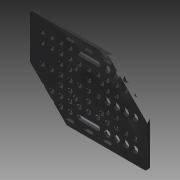
# Autodesk Inventor part: 80mm gantry plate
Saved by Autodesk Inventor 2014 SP1 (Build 180222100, 222)
## iProperties
Created: 2016-04-10
Part Number: 80mm gantry plate
Material: Generic
Document SubType Name: Modeling
Designer: Ben
Density: 1 g/cm^3
Appearance: Default
Author: Ben
Autodesk Inventor part; units mm, degrees
ref_plane "YZ Plane" through (0, 0, 0) normal (1, 0, 0) x (0, 1, 0)
ref_plane "XZ Plane" through (0, 0, 0) normal (0, 1, 0) x (-1, 0, 0)
ref_plane "XY Plane" through (0, 0, 0) normal (0, 0, 1) x (1, 0, 0)
sketch "Sketch1" plane through (0, 0, 0) normal (0, 0, 1) x (1, 0, 0)
  line L0 (-63.5, 44) -> (63.5, 44)
  line L1 (63.5, 44) -> (63.5, -44)
  line L2 (63.5, -44) -> (-63.5, -44)
  line L3 (-63.5, -44) -> (-63.5, 44)
  line L4 (0, 44) -> (0, -44) construction
  line L5 (-63.5, 0) -> (63.5, 0) construction
  point P0 (0, 0)
  dimension "d0" = 127
  dimension "d1" = 88
  constraints: 12 end point, 6 midpoint, 2 parallel, 1 horizontal, 1 perpendicular
  measures "d0" distance of L1.end L2.end
  measures "d1" distance of L0.end L1.end
extrude "Extrusion1" add sketch "Sketch1" along normal blind 3
sketch "Sketch2" plane through (0, 0, 3) normal (0, 0, 1) x (1, 0, 0)
  line L0 (-63.5, -44) -> (63.5, -44) projected
  line L1 (63.5, -44) -> (63.5, 44) projected
  circle A0 centre (0, 0) radius 2.5
  line L2 (0, 0) -> (78.1267, 0) construction
  line L3 (0, 0) -> (0, 59.5743) construction
  circle A1 centre (10, 0) radius 2.5
  circle A2 centre (20, 0) radius 2.5
  circle A3 centre (30, 0) radius 2.5
  circle A4 centre (40, 0) radius 2.5
  circle A5 centre (50, 0) radius 2.5
  circle A6 centre (-10, 0) radius 2.5
  circle A7 centre (0, 0) radius 2.5
  circle A8 centre (10, 0) radius 2.5
  circle A9 centre (20, 0) radius 2.5
  circle A10 centre (30, 0) radius 2.5
  circle A11 centre (40, 0) radius 2.5
  circle A12 centre (-20, 0) radius 2.5
  circle A13 centre (-10, 0) radius 2.5
  circle A14 centre (0, 0) radius 2.5
  circle A15 centre (10, 0) radius 2.5
  circle A16 centre (20, 0) radius 2.5
  circle A17 centre (30, 0) radius 2.5
  circle A18 centre (-30, 0) radius 2.5
  circle A19 centre (-20, 0) radius 2.5
  circle A20 centre (-10, 0) radius 2.5
  circle A21 centre (0, 0) radius 2.5
  circle A22 centre (10, 0) radius 2.5
  circle A23 centre (20, 0) radius 2.5
  circle A24 centre (-40, 0) radius 2.5
  circle A25 centre (-30, 0) radius 2.5
  circle A26 centre (-20, 0) radius 2.5
  circle A27 centre (-10, 0) radius 2.5
  circle A28 centre (0, 0) radius 2.5
  circle A29 centre (10, 0) radius 2.5
  circle A30 centre (-50, 0) radius 2.5
  circle A31 centre (-40, 0) radius 2.5
  circle A32 centre (-30, 0) radius 2.5
  circle A33 centre (-20, 0) radius 2.5
  circle A34 centre (-10, 0) radius 2.5
  circle A35 centre (0, 0) radius 2.5
  circle A36 centre (0, 20) radius 2.5
  circle A37 centre (10, 20) radius 2.5
  circle A38 centre (20, 20) radius 2.5
  circle A39 centre (30, 20) radius 2.5
  circle A40 centre (40, 20) radius 2.5
  circle A41 centre (50, 20) radius 2.5
  circle A42 centre (-10, 20) radius 2.5
  circle A43 centre (0, 20) radius 2.5
  circle A44 centre (10, 20) radius 2.5
  circle A45 centre (20, 20) radius 2.5
  circle A46 centre (30, 20) radius 2.5
  circle A47 centre (40, 20) radius 2.5
  circle A48 centre (-20, 20) radius 2.5
  circle A49 centre (-10, 20) radius 2.5
  circle A50 centre (0, 20) radius 2.5
  circle A51 centre (10, 20) radius 2.5
  circle A52 centre (20, 20) radius 2.5
  circle A53 centre (30, 20) radius 2.5
  circle A54 centre (-30, 20) radius 2.5
  circle A55 centre (-20, 20) radius 2.5
  circle A56 centre (-10, 20) radius 2.5
  circle A57 centre (0, 20) radius 2.5
  circle A58 centre (10, 20) radius 2.5
  circle A59 centre (20, 20) radius 2.5
  circle A60 centre (-40, 20) radius 2.5
  circle A61 centre (-30, 20) radius 2.5
  circle A62 centre (-20, 20) radius 2.5
  circle A63 centre (-10, 20) radius 2.5
  circle A64 centre (0, 20) radius 2.5
  circle A65 centre (10, 20) radius 2.5
  circle A66 centre (-50, 20) radius 2.5
  circle A67 centre (-40, 20) radius 2.5
  circle A68 centre (-30, 20) radius 2.5
  circle A69 centre (-20, 20) radius 2.5
  circle A70 centre (-10, 20) radius 2.5
  circle A71 centre (0, 20) radius 2.5
  circle A72 centre (0, -20) radius 2.5
  circle A73 centre (10, -20) radius 2.5
  circle A74 centre (20, -20) radius 2.5
  circle A75 centre (30, -20) radius 2.5
  circle A76 centre (40, -20) radius 2.5
  circle A77 centre (50, -20) radius 2.5
  circle A78 centre (-10, -20) radius 2.5
  circle A79 centre (0, -20) radius 2.5
  circle A80 centre (10, -20) radius 2.5
  circle A81 centre (20, -20) radius 2.5
  circle A82 centre (30, -20) radius 2.5
  circle A83 centre (40, -20) radius 2.5
  circle A84 centre (-20, -20) radius 2.5
  circle A85 centre (-10, -20) radius 2.5
  circle A86 centre (0, -20) radius 2.5
  circle A87 centre (10, -20) radius 2.5
  circle A88 centre (20, -20) radius 2.5
  circle A89 centre (30, -20) radius 2.5
  circle A90 centre (-30, -20) radius 2.5
  circle A91 centre (-20, -20) radius 2.5
  circle A92 centre (-10, -20) radius 2.5
  circle A93 centre (0, -20) radius 2.5
  circle A94 centre (10, -20) radius 2.5
  circle A95 centre (20, -20) radius 2.5
  circle A96 centre (-40, -20) radius 2.5
  circle A97 centre (-30, -20) radius 2.5
  circle A98 centre (-20, -20) radius 2.5
  circle A99 centre (-10, -20) radius 2.5
  circle A100 centre (0, -20) radius 2.5
  circle A101 centre (10, -20) radius 2.5
  circle A102 centre (-50, -20) radius 2.5
  circle A103 centre (-40, -20) radius 2.5
  circle A104 centre (-30, -20) radius 2.5
  circle A105 centre (-20, -20) radius 2.5
  circle A106 centre (-10, -20) radius 2.5
  circle A107 centre (0, -20) radius 2.5
  circle A108 centre (0, 0) radius 2.5
  circle A109 centre (10, 0) radius 2.5
  circle A110 centre (20, 0) radius 2.5
  circle A111 centre (30, 0) radius 2.5
  circle A112 centre (40, 0) radius 2.5
  circle A113 centre (50, 0) radius 2.5
  circle A114 centre (-10, 0) radius 2.5
  circle A115 centre (0, 0) radius 2.5
  circle A116 centre (10, 0) radius 2.5
  circle A117 centre (20, 0) radius 2.5
  circle A118 centre (30, 0) radius 2.5
  circle A119 centre (40, 0) radius 2.5
  circle A120 centre (-20, 0) radius 2.5
  circle A121 centre (-10, 0) radius 2.5
  circle A122 centre (0, 0) radius 2.5
  circle A123 centre (10, 0) radius 2.5
  circle A124 centre (20, 0) radius 2.5
  circle A125 centre (30, 0) radius 2.5
  circle A126 centre (-30, 0) radius 2.5
  circle A127 centre (-20, 0) radius 2.5
  circle A128 centre (-10, 0) radius 2.5
  circle A129 centre (0, 0) radius 2.5
  circle A130 centre (10, 0) radius 2.5
  circle A131 centre (20, 0) radius 2.5
  circle A132 centre (-40, 0) radius 2.5
  circle A133 centre (-30, 0) radius 2.5
  circle A134 centre (-20, 0) radius 2.5
  circle A135 centre (-10, 0) radius 2.5
  circle A136 centre (0, 0) radius 2.5
  circle A137 centre (10, 0) radius 2.5
  circle A138 centre (-50, 0) radius 2.5
  circle A139 centre (-40, 0) radius 2.5
  circle A140 centre (-30, 0) radius 2.5
  circle A141 centre (-20, 0) radius 2.5
  circle A142 centre (-10, 0) radius 2.5
  circle A143 centre (0, 0) radius 2.5
  circle A144 centre (-14.1421, -14.1421) radius 2.5
  circle A145 centre (0, -20) radius 2.5
  circle A146 centre (14.1421, -14.1421) radius 2.5
  circle A147 centre (20, 0) radius 2.5
  circle A148 centre (14.1421, 14.1421) radius 2.5
  circle A149 centre (0, 20) radius 2.5
  circle A150 centre (-14.1421, 14.1421) radius 2.5
  circle A151 centre (0, -10) radius 2.5
  circle A152 centre (10, 0) radius 2.5
  circle A153 centre (0, 10) radius 2.5
  circle A154 centre (-20, 10) radius 2.5
  circle A155 centre (-30, 10) radius 2.5
  circle A156 centre (-20, 10) radius 2.5
  circle A157 centre (-30, 10) radius 2.5
  circle A158 centre (-20, 10) radius 2.5
  circle A159 centre (-30, 10) radius 2.5
  circle A160 centre (-20, 10) radius 2.5
  circle A161 centre (-20, 10) radius 2.5
  circle A162 centre (-30, 10) radius 2.5
  circle A163 centre (-20, 10) radius 2.5
  circle A164 centre (-20, 10) radius 2.5
  circle A165 centre (-20, 10) radius 2.5
  circle A166 centre (-30, 10) radius 2.5
  circle A167 centre (-30, 10) radius 2.5
  circle A168 centre (-20, 20) radius 2.5
  circle A169 centre (-30, 20) radius 2.5
  circle A170 centre (-20, 20) radius 2.5
  circle A171 centre (-30, 20) radius 2.5
  circle A172 centre (-20, 20) radius 2.5
  circle A173 centre (-30, 20) radius 2.5
  circle A174 centre (-20, 20) radius 2.5
  circle A175 centre (-20, 20) radius 2.5
  circle A176 centre (-30, 20) radius 2.5
  circle A177 centre (-20, 20) radius 2.5
  circle A178 centre (-20, 20) radius 2.5
  circle A179 centre (-20, 20) radius 2.5
  circle A180 centre (-30, 20) radius 2.5
  circle A181 centre (-30, 20) radius 2.5
  circle A182 centre (-20, 30) radius 2.5
  circle A183 centre (-30, 30) radius 2.5
  circle A184 centre (-20, 30) radius 2.5
  circle A185 centre (-30, 30) radius 2.5
  circle A186 centre (-20, 30) radius 2.5
  circle A187 centre (-30, 30) radius 2.5
  circle A188 centre (-20, 30) radius 2.5
  circle A189 centre (-20, 30) radius 2.5
  circle A190 centre (-30, 30) radius 2.5
  circle A191 centre (-20, 30) radius 2.5
  circle A192 centre (-20, 30) radius 2.5
  circle A193 centre (-20, 30) radius 2.5
  circle A194 centre (-30, 30) radius 2.5
  circle A195 centre (-30, 30) radius 2.5
  circle A196 centre (-20, -10) radius 2.5
  circle A197 centre (-30, -10) radius 2.5
  circle A198 centre (-20, -10) radius 2.5
  circle A199 centre (-30, -10) radius 2.5
  circle A200 centre (-20, -10) radius 2.5
  circle A201 centre (-30, -10) radius 2.5
  circle A202 centre (-20, -10) radius 2.5
  circle A203 centre (-20, -10) radius 2.5
  circle A204 centre (-30, -10) radius 2.5
  circle A205 centre (-20, -10) radius 2.5
  circle A206 centre (-20, -10) radius 2.5
  circle A207 centre (-20, -10) radius 2.5
  circle A208 centre (-30, -10) radius 2.5
  circle A209 centre (-30, -10) radius 2.5
  circle A210 centre (-20, 0) radius 2.5
  circle A211 centre (-30, 0) radius 2.5
  circle A212 centre (-20, 0) radius 2.5
  circle A213 centre (-30, 0) radius 2.5
  circle A214 centre (-20, 0) radius 2.5
  circle A215 centre (-30, 0) radius 2.5
  circle A216 centre (-20, 0) radius 2.5
  circle A217 centre (-20, 0) radius 2.5
  circle A218 centre (-30, 0) radius 2.5
  circle A219 centre (-20, 0) radius 2.5
  circle A220 centre (-20, 0) radius 2.5
  circle A221 centre (-20, 0) radius 2.5
  circle A222 centre (-30, 0) radius 2.5
  circle A223 centre (-30, 0) radius 2.5
  circle A224 centre (-20, 10) radius 2.5
  circle A225 centre (-30, 10) radius 2.5
  circle A226 centre (-20, 10) radius 2.5
  circle A227 centre (-30, 10) radius 2.5
  circle A228 centre (-20, 10) radius 2.5
  circle A229 centre (-30, 10) radius 2.5
  circle A230 centre (-20, 10) radius 2.5
  circle A231 centre (-20, 10) radius 2.5
  circle A232 centre (-30, 10) radius 2.5
  circle A233 centre (-20, 10) radius 2.5
  circle A234 centre (-20, 10) radius 2.5
  circle A235 centre (-20, 10) radius 2.5
  circle A236 centre (-30, 10) radius 2.5
  circle A237 centre (-30, 10) radius 2.5
  circle A238 centre (-20, 20) radius 2.5
  circle A239 centre (-30, 20) radius 2.5
  circle A240 centre (-20, 20) radius 2.5
  circle A241 centre (-30, 20) radius 2.5
  circle A242 centre (-20, 20) radius 2.5
  circle A243 centre (-30, 20) radius 2.5
  circle A244 centre (-20, 20) radius 2.5
  circle A245 centre (-20, 20) radius 2.5
  circle A246 centre (-30, 20) radius 2.5
  circle A247 centre (-20, 20) radius 2.5
  circle A248 centre (-20, 20) radius 2.5
  circle A249 centre (-20, 20) radius 2.5
  circle A250 centre (-30, 20) radius 2.5
  circle A251 centre (-30, 20) radius 2.5
  circle A252 centre (-20, -20) radius 2.5
  circle A253 centre (-30, -20) radius 2.5
  circle A254 centre (-20, -20) radius 2.5
  circle A255 centre (-30, -20) radius 2.5
  circle A256 centre (-20, -20) radius 2.5
  circle A257 centre (-30, -20) radius 2.5
  circle A258 centre (-20, -20) radius 2.5
  circle A259 centre (-20, -20) radius 2.5
  circle A260 centre (-30, -20) radius 2.5
  circle A261 centre (-20, -20) radius 2.5
  circle A262 centre (-20, -20) radius 2.5
  circle A263 centre (-20, -20) radius 2.5
  circle A264 centre (-30, -20) radius 2.5
  circle A265 centre (-30, -20) radius 2.5
  circle A266 centre (-20, -10) radius 2.5
  circle A267 centre (-30, -10) radius 2.5
  circle A268 centre (-20, -10) radius 2.5
  circle A269 centre (-30, -10) radius 2.5
  circle A270 centre (-20, -10) radius 2.5
  circle A271 centre (-30, -10) radius 2.5
  circle A272 centre (-20, -10) radius 2.5
  circle A273 centre (-20, -10) radius 2.5
  circle A274 centre (-30, -10) radius 2.5
  circle A275 centre (-20, -10) radius 2.5
  circle A276 centre (-20, -10) radius 2.5
  circle A277 centre (-20, -10) radius 2.5
  circle A278 centre (-30, -10) radius 2.5
  circle A279 centre (-30, -10) radius 2.5
  circle A280 centre (-20, 0) radius 2.5
  circle A281 centre (-30, 0) radius 2.5
  circle A282 centre (-20, 0) radius 2.5
  circle A283 centre (-30, 0) radius 2.5
  circle A284 centre (-20, 0) radius 2.5
  circle A285 centre (-30, 0) radius 2.5
  circle A286 centre (-20, 0) radius 2.5
  circle A287 centre (-20, 0) radius 2.5
  circle A288 centre (-30, 0) radius 2.5
  circle A289 centre (-20, 0) radius 2.5
  circle A290 centre (-20, 0) radius 2.5
  circle A291 centre (-20, 0) radius 2.5
  circle A292 centre (-30, 0) radius 2.5
  circle A293 centre (-30, 0) radius 2.5
  circle A294 centre (-20, 10) radius 2.5
  circle A295 centre (-30, 10) radius 2.5
  circle A296 centre (-20, 10) radius 2.5
  circle A297 centre (-30, 10) radius 2.5
  circle A298 centre (-20, 10) radius 2.5
  circle A299 centre (-30, 10) radius 2.5
  circle A300 centre (-20, 10) radius 2.5
  circle A301 centre (-20, 10) radius 2.5
  circle A302 centre (-30, 10) radius 2.5
  circle A303 centre (-20, 10) radius 2.5
  circle A304 centre (-20, 10) radius 2.5
  circle A305 centre (-20, 10) radius 2.5
  circle A306 centre (-30, 10) radius 2.5
  circle A307 centre (-30, 10) radius 2.5
  circle A308 centre (-20, -30) radius 2.5
  circle A309 centre (-30, -30) radius 2.5
  circle A310 centre (-20, -30) radius 2.5
  circle A311 centre (-30, -30) radius 2.5
  circle A312 centre (-20, -30) radius 2.5
  circle A313 centre (-30, -30) radius 2.5
  circle A314 centre (-20, -30) radius 2.5
  circle A315 centre (-20, -30) radius 2.5
  circle A316 centre (-30, -30) radius 2.5
  circle A317 centre (-20, -30) radius 2.5
  circle A318 centre (-20, -30) radius 2.5
  circle A319 centre (-20, -30) radius 2.5
  circle A320 centre (-30, -30) radius 2.5
  circle A321 centre (-30, -30) radius 2.5
  circle A322 centre (-20, -20) radius 2.5
  circle A323 centre (-30, -20) radius 2.5
  circle A324 centre (-20, -20) radius 2.5
  circle A325 centre (-30, -20) radius 2.5
  circle A326 centre (-20, -20) radius 2.5
  circle A327 centre (-30, -20) radius 2.5
  circle A328 centre (-20, -20) radius 2.5
  circle A329 centre (-20, -20) radius 2.5
  circle A330 centre (-30, -20) radius 2.5
  circle A331 centre (-20, -20) radius 2.5
  circle A332 centre (-20, -20) radius 2.5
  circle A333 centre (-20, -20) radius 2.5
  circle A334 centre (-30, -20) radius 2.5
  circle A335 centre (-30, -20) radius 2.5
  circle A336 centre (-20, -10) radius 2.5
  circle A337 centre (-30, -10) radius 2.5
  circle A338 centre (-20, -10) radius 2.5
  circle A339 centre (-30, -10) radius 2.5
  circle A340 centre (-20, -10) radius 2.5
  circle A341 centre (-30, -10) radius 2.5
  circle A342 centre (-20, -10) radius 2.5
  circle A343 centre (-20, -10) radius 2.5
  circle A344 centre (-30, -10) radius 2.5
  circle A345 centre (-20, -10) radius 2.5
  circle A346 centre (-20, -10) radius 2.5
  circle A347 centre (-20, -10) radius 2.5
  circle A348 centre (-30, -10) radius 2.5
  circle A349 centre (-30, -10) radius 2.5
  circle A350 centre (-20, 0) radius 2.5
  circle A351 centre (-30, 0) radius 2.5
  circle A352 centre (-20, 0) radius 2.5
  circle A353 centre (-30, 0) radius 2.5
  circle A354 centre (-20, 0) radius 2.5
  circle A355 centre (-30, 0) radius 2.5
  circle A356 centre (-20, 0) radius 2.5
  circle A357 centre (-20, 0) radius 2.5
  circle A358 centre (-30, 0) radius 2.5
  circle A359 centre (-20, 0) radius 2.5
  circle A360 centre (-20, 0) radius 2.5
  circle A361 centre (-20, 0) radius 2.5
  circle A362 centre (-30, 0) radius 2.5
  circle A363 centre (-30, 0) radius 2.5
  circle A364 centre (-40, 30) radius 2.5
  circle A365 centre (-40, 30) radius 2.5
  circle A366 centre (-40, 30) radius 2.5
  circle A367 centre (-40, 30) radius 2.5
  circle A368 centre (-40, 30) radius 2.5
  circle A369 centre (-40, 30) radius 2.5
  circle A370 centre (-40, 30) radius 2.5
  circle A371 centre (-40, 30) radius 2.5
  circle A372 centre (-50, 30) radius 2.5
  circle A373 centre (-50, 30) radius 2.5
  circle A374 centre (-50, 30) radius 2.5
  circle A375 centre (-50, 30) radius 2.5
  circle A376 centre (-50, 30) radius 2.5
  circle A377 centre (-50, 30) radius 2.5
  circle A378 centre (-40, -30) radius 2.5
  circle A379 centre (-40, -30) radius 2.5
  circle A380 centre (-40, -30) radius 2.5
  circle A381 centre (-40, -30) radius 2.5
  circle A382 centre (-40, -30) radius 2.5
  circle A383 centre (-40, -30) radius 2.5
  circle A384 centre (-40, -30) radius 2.5
  circle A385 centre (-40, -30) radius 2.5
  circle A386 centre (-50, -30) radius 2.5
  circle A387 centre (-50, -30) radius 2.5
  circle A388 centre (-50, -30) radius 2.5
  circle A389 centre (-50, -30) radius 2.5
  circle A390 centre (-50, -30) radius 2.5
  circle A391 centre (-50, -30) radius 2.5
  circle A392 centre (20, 10) radius 2.5
  circle A393 centre (20, 10) radius 2.5
  circle A394 centre (20, 10) radius 2.5
  circle A395 centre (20, 10) radius 2.5
  circle A396 centre (20, 10) radius 2.5
  circle A397 centre (20, 10) radius 2.5
  circle A398 centre (20, 10) radius 2.5
  circle A399 centre (20, 10) radius 2.5
  circle A400 centre (30, 10) radius 2.5
  circle A401 centre (30, 10) radius 2.5
  circle A402 centre (30, 10) radius 2.5
  circle A403 centre (30, 10) radius 2.5
  circle A404 centre (30, 10) radius 2.5
  circle A405 centre (30, 10) radius 2.5
  circle A406 centre (20, 30) radius 2.5
  circle A407 centre (20, 30) radius 2.5
  circle A408 centre (20, 30) radius 2.5
  circle A409 centre (20, 30) radius 2.5
  circle A410 centre (20, 30) radius 2.5
  circle A411 centre (20, 30) radius 2.5
  circle A412 centre (20, 30) radius 2.5
  circle A413 centre (20, 30) radius 2.5
  circle A414 centre (30, 30) radius 2.5
  circle A415 centre (30, 30) radius 2.5
  circle A416 centre (30, 30) radius 2.5
  circle A417 centre (30, 30) radius 2.5
  circle A418 centre (30, 30) radius 2.5
  circle A419 centre (30, 30) radius 2.5
  circle A420 centre (20, -10) radius 2.5
  circle A421 centre (20, -10) radius 2.5
  circle A422 centre (20, -10) radius 2.5
  circle A423 centre (20, -10) radius 2.5
  circle A424 centre (20, -10) radius 2.5
  circle A425 centre (20, -10) radius 2.5
  circle A426 centre (20, -10) radius 2.5
  circle A427 centre (20, -10) radius 2.5
  circle A428 centre (30, -10) radius 2.5
  circle A429 centre (30, -10) radius 2.5
  circle A430 centre (30, -10) radius 2.5
  circle A431 centre (30, -10) radius 2.5
  circle A432 centre (30, -10) radius 2.5
  circle A433 centre (30, -10) radius 2.5
  circle A434 centre (20, 10) radius 2.5
  circle A435 centre (20, 10) radius 2.5
  circle A436 centre (20, 10) radius 2.5
  circle A437 centre (20, 10) radius 2.5
  circle A438 centre (20, 10) radius 2.5
  circle A439 centre (20, 10) radius 2.5
  circle A440 centre (20, 10) radius 2.5
  circle A441 centre (20, 10) radius 2.5
  circle A442 centre (30, 10) radius 2.5
  circle A443 centre (30, 10) radius 2.5
  circle A444 centre (30, 10) radius 2.5
  circle A445 centre (30, 10) radius 2.5
  circle A446 centre (30, 10) radius 2.5
  circle A447 centre (30, 10) radius 2.5
  circle A448 centre (20, -10) radius 2.5
  circle A449 centre (20, -10) radius 2.5
  circle A450 centre (20, -10) radius 2.5
  circle A451 centre (20, -10) radius 2.5
  circle A452 centre (20, -10) radius 2.5
  circle A453 centre (20, -10) radius 2.5
  circle A454 centre (20, -10) radius 2.5
  circle A455 centre (20, -10) radius 2.5
  circle A456 centre (30, -10) radius 2.5
  circle A457 centre (30, -10) radius 2.5
  circle A458 centre (30, -10) radius 2.5
  circle A459 centre (30, -10) radius 2.5
  circle A460 centre (30, -10) radius 2.5
  circle A461 centre (30, -10) radius 2.5
  circle A462 centre (20, 10) radius 2.5
  circle A463 centre (20, 10) radius 2.5
  circle A464 centre (20, 10) radius 2.5
  circle A465 centre (20, 10) radius 2.5
  circle A466 centre (20, 10) radius 2.5
  circle A467 centre (20, 10) radius 2.5
  circle A468 centre (20, 10) radius 2.5
  circle A469 centre (20, 10) radius 2.5
  circle A470 centre (30, 10) radius 2.5
  circle A471 centre (30, 10) radius 2.5
  circle A472 centre (30, 10) radius 2.5
  circle A473 centre (30, 10) radius 2.5
  circle A474 centre (30, 10) radius 2.5
  circle A475 centre (30, 10) radius 2.5
  circle A476 centre (20, -30) radius 2.5
  circle A477 centre (20, -30) radius 2.5
  circle A478 centre (20, -30) radius 2.5
  circle A479 centre (20, -30) radius 2.5
  circle A480 centre (20, -30) radius 2.5
  circle A481 centre (20, -30) radius 2.5
  circle A482 centre (20, -30) radius 2.5
  circle A483 centre (20, -30) radius 2.5
  circle A484 centre (30, -30) radius 2.5
  circle A485 centre (30, -30) radius 2.5
  circle A486 centre (30, -30) radius 2.5
  circle A487 centre (30, -30) radius 2.5
  circle A488 centre (30, -30) radius 2.5
  circle A489 centre (30, -30) radius 2.5
  circle A490 centre (20, -10) radius 2.5
  circle A491 centre (20, -10) radius 2.5
  circle A492 centre (20, -10) radius 2.5
  circle A493 centre (20, -10) radius 2.5
  circle A494 centre (20, -10) radius 2.5
  circle A495 centre (20, -10) radius 2.5
  circle A496 centre (20, -10) radius 2.5
  circle A497 centre (20, -10) radius 2.5
  circle A498 centre (30, -10) radius 2.5
  circle A499 centre (30, -10) radius 2.5
  circle A500 centre (30, -10) radius 2.5
  circle A501 centre (30, -10) radius 2.5
  circle A502 centre (30, -10) radius 2.5
  circle A503 centre (30, -10) radius 2.5
  circle A504 centre (50, 30) radius 2.5
  circle A505 centre (50, 30) radius 2.5
  circle A506 centre (50, 30) radius 2.5
  circle A507 centre (50, 30) radius 2.5
  circle A508 centre (50, 30) radius 2.5
  circle A509 centre (50, 30) radius 2.5
  circle A510 centre (40, 30) radius 2.5
  circle A511 centre (40, 30) radius 2.5
  circle A512 centre (40, 30) radius 2.5
  circle A513 centre (40, 30) radius 2.5
  circle A514 centre (40, 30) radius 2.5
  circle A515 centre (40, 30) radius 2.5
  circle A516 centre (40, 30) radius 2.5
  circle A517 centre (40, 30) radius 2.5
  circle A518 centre (40, -30) radius 2.5
  circle A519 centre (40, -30) radius 2.5
  circle A520 centre (40, -30) radius 2.5
  circle A521 centre (40, -30) radius 2.5
  circle A522 centre (40, -30) radius 2.5
  circle A523 centre (40, -30) radius 2.5
  circle A524 centre (40, -30) radius 2.5
  circle A525 centre (40, -30) radius 2.5
  circle A526 centre (50, -30) radius 2.5
  circle A527 centre (50, -30) radius 2.5
  circle A528 centre (50, -30) radius 2.5
  circle A529 centre (50, -30) radius 2.5
  circle A530 centre (50, -30) radius 2.5
  circle A531 centre (50, -30) radius 2.5
  dimension "d4" = 5
  dimension "d7" = 10
  dimension "d10" = 10
  dimension "d15" = 20
  dimension "d18" = 20
  dimension "d23" = 360
  dimension "d27" = 360
  dimension "d31" = 10
  dimension "d34" = 10
  dimension "d39" = 20
  constraints: 532 centre point, 140 symmetric about line, 4 coincident, 4 end point, 4 vertical, 3 horizontal, 2 perpendicular, 931 other
  measures "d4" diameter of A0
  measures "d7" distance of L2.start A1.centre
  measures "d10" distance of L2.start A6.centre
  measures "d15" distance of A6.centre A42.centre
  measures "d18" distance of A6.centre A78.centre
  measures "d31" distance of A12.centre A154.centre
  measures "d34" distance of A12.centre A196.centre
  measures "d39" distance of A183.centre A372.centre
extrude "Extrusion2" cut sketch "Sketch2" against normal up to next
sketch "Sketch3" plane through (0, 0, 3) normal (0, 0, 1) x (1, 0, 0)
  circle A0 centre (-50, 30) radius 2.5 projected
  circle A1 centre (10, 20) radius 2.5 projected
  circle A2 centre (-10, 20) radius 2.5 projected
  circle A3 centre (0, 0) radius 2.5 projected
  line L0 (63.5, 44) -> (-63.5, 44) projected
  line L1 (-63.5, 44) -> (-63.5, -44) projected
  line L2 (-63.5, -44) -> (63.5, -44) projected
  line L3 (63.5, -44) -> (63.5, 44) projected
  line L4 (-10, 30) -> (10, 30) construction
  line L5 (-10, 32.5) -> (10, 32.5)
  line L6 (10, 27.5) -> (-10, 27.5)
  arc A4 (-10, 32.5) -> (-10, 27.5) centre (-10, 30) ccw
  arc A5 (10, 27.5) -> (10, 32.5) centre (10, 30) ccw
  line L7 (-10, 44) -> (-10, -44) construction
  line L8 (10, 44) -> (10, -44) construction
  line L9 (-63.5, 30) -> (63.5, 30) construction
  line L10 (0, 0) -> (73.5761, 0) construction
  line L11 (-10, -30) -> (10, -30) construction
  line L12 (-10, -32.5) -> (10, -32.5)
  line L13 (10, -27.5) -> (-10, -27.5)
  arc A6 (-10, -27.5) -> (-10, -32.5) centre (-10, -30) ccw
  arc A7 (10, -32.5) -> (10, -27.5) centre (10, -30) ccw
  line L14 (-3.25, -37.7) -> (3.25, -37.7) construction
  line L15 (-3.25, -39.2) -> (3.25, -39.2)
  line L16 (3.25, -36.2) -> (-3.25, -36.2)
  arc A8 (-3.25, -36.2) -> (-3.25, -39.2) centre (-3.25, -37.7) ccw
  arc A9 (3.25, -39.2) -> (3.25, -36.2) centre (3.25, -37.7) ccw
  line L17 (0, 0) -> (0, -48.0839) construction
  line L18 (-23.4, -37.7) -> (-16.9, -37.7) construction
  line L19 (-23.4, -39.2) -> (-16.9, -39.2)
  line L20 (-16.9, -36.2) -> (-23.4, -36.2)
  arc A10 (-23.4, -36.2) -> (-23.4, -39.2) centre (-23.4, -37.7) ccw
  arc A11 (-16.9, -39.2) -> (-16.9, -36.2) centre (-16.9, -37.7) ccw
  line L21 (16.9, -37.7) -> (23.4, -37.7) construction
  line L22 (16.9, -39.2) -> (23.4, -39.2)
  line L23 (23.4, -36.2) -> (16.9, -36.2)
  arc A12 (16.9, -36.2) -> (16.9, -39.2) centre (16.9, -37.7) ccw
  arc A13 (23.4, -39.2) -> (23.4, -36.2) centre (23.4, -37.7) ccw
  line L24 (-3.25, -37.7) -> (3.25, -37.7) construction
  line L25 (-3.25, -39.2) -> (3.25, -39.2)
  line L26 (3.25, -36.2) -> (-3.25, -36.2)
  arc A14 (-3.25, -36.2) -> (-3.25, -39.2) centre (-3.25, -37.7) ccw
  arc A15 (3.25, -39.2) -> (3.25, -36.2) centre (3.25, -37.7) ccw
  line L27 (-3.25, 37.7) -> (3.25, 37.7) construction
  line L28 (-3.25, 39.2) -> (3.25, 39.2)
  line L29 (3.25, 36.2) -> (-3.25, 36.2)
  arc A16 (-3.25, 39.2) -> (-3.25, 36.2) centre (-3.25, 37.7) ccw
  arc A17 (3.25, 36.2) -> (3.25, 39.2) centre (3.25, 37.7) ccw
  arc A18 (-23.4, 39.2) -> (-23.4, 36.2) centre (-23.4, 37.7) ccw
  line L30 (-16.9, 36.2) -> (-23.4, 36.2)
  line L31 (-23.4, 37.7) -> (-16.9, 37.7) construction
  line L32 (-23.4, 39.2) -> (-16.9, 39.2)
  arc A19 (-16.9, 36.2) -> (-16.9, 39.2) centre (-16.9, 37.7) ccw
  arc A20 (16.9, 39.2) -> (16.9, 36.2) centre (16.9, 37.7) ccw
  line L33 (23.4, 36.2) -> (16.9, 36.2)
  line L34 (16.9, 37.7) -> (23.4, 37.7) construction
  line L35 (16.9, 39.2) -> (23.4, 39.2)
  arc A21 (23.4, 36.2) -> (23.4, 39.2) centre (23.4, 37.7) ccw
  arc A22 (-3.25, 39.2) -> (-3.25, 36.2) centre (-3.25, 37.7) ccw
  line L36 (3.25, 36.2) -> (-3.25, 36.2)
  line L37 (-3.25, 37.7) -> (3.25, 37.7) construction
  line L38 (-3.25, 39.2) -> (3.25, 39.2)
  arc A23 (3.25, 36.2) -> (3.25, 39.2) centre (3.25, 37.7) ccw
  point P0 (0, 30)
  point P1 (0, 30)
  point P2 (0, -30)
  point P3 (0, -30)
  point P4 (0, -37.7)
  point P5 (-20.15, -37.7)
  point P6 (20.15, -37.7)
  point P7 (0, -37.7)
  point P8 (0, 37.7)
  point P9 (-20.15, 37.7)
  point P10 (20.15, 37.7)
  point P11 (0, 37.7)
  dimension "d46" = 5
  dimension "d47" = 6.5
  dimension "d48" = 3
  dimension "d49" = 7.7
  dimension "d52" = 20.15
  dimension "d55" = 20.15
  constraints: 90 end point, 40 point on circle, 36 symmetric about line, 20 centre point, 12 point on line, 8 tangent, 5 midpoint, 5 parallel, 4 perpendicular, 2 horizontal, 46 other
  measures "d46" distance between parallel lines of L6 L5
  measures "d47" distance of L14.start L14.end
  measures "d48" diameter of A9
  measures "d49" distance between parallel lines of L11 L14
  measures "d52" distance of L16.end L20.end
  measures "d55" distance of L16.end L23.end
extrude "Extrusion3" cut sketch "Sketch3" against normal up to next contours L5 A5 L6 A4 | A6 L13 A7 L12 | A8 L16 A9 L15 | A10 L20 A11 L19 | A12 L23 A13 L22 | L28 A17 L29 A16 | L32 A19 L30 A18 | L35 A21 L33 A20
fillet "Fillet1" radius 3.38 4 edges at (63.5, -44, 1.5) (-63.5, -44, 1.5) (63.5, 44, 1.5) (-63.5, 44, 1.5)
sketch "Sketch4" plane through (0, 0, 3) normal (0, 0, 1) x (1, 0, 0)
  line L0 (-60.12, -44) -> (60.12, -44) projected
  line L1 (63.5, -40.62) -> (63.5, 40.62) projected
  circle A0 centre (50, -30) radius 2.5 projected
  circle A1 centre (30, -30) radius 2.5 projected
  circle A2 centre (40, 30) radius 2.5 projected
  circle A3 centre (20, 30) radius 2.5 projected
  circle A4 centre (50, 0) radius 2.5 projected
  circle A5 centre (30, 0) radius 2.5 projected
  circle A6 centre (20, 0) radius 2.5 projected
  circle A7 centre (40, 0) radius 2.5 projected
  circle A8 centre (30, 30) radius 2.5 projected
  circle A9 centre (50, 30) radius 2.5 projected
  circle A10 centre (40, -30) radius 2.5 projected
  circle A11 centre (20, -30) radius 2.5 projected
  circle A12 centre (20, 0) radius 3.6
  circle A13 centre (30, 0) radius 3.6
  circle A14 centre (40, 0) radius 3.6
  circle A15 centre (50, 0) radius 3.6
  circle A16 centre (20, 30) radius 3.6
  circle A17 centre (30, 30) radius 3.6
  circle A18 centre (40, 30) radius 3.6
  circle A19 centre (50, 30) radius 3.6
  circle A20 centre (20, -30) radius 3.6
  circle A21 centre (30, -30) radius 3.6
  circle A22 centre (40, -30) radius 3.6
  circle A23 centre (50, -30) radius 3.6
  circle A24 centre (20, 0) radius 3.6
  circle A25 centre (30, 0) radius 3.6
  circle A26 centre (40, 0) radius 3.6
  circle A27 centre (50, 0) radius 3.6
  dimension "d61" = 7.2
  dimension "d64" = 10
  dimension "d71" = 30
  dimension "d74" = 30
  constraints: 16 centre point, 2 vertical, 1 coincident, 1 horizontal, 30 other
  measures "d61" diameter of A12
  measures "d64" distance of A12.centre A13.centre
  measures "d71" distance of A15.centre A19.centre
  measures "d74" distance of A15.centre A23.centre
extrude "Extrusion4" cut sketch "Sketch4" against normal up to next
body "Solid1"
